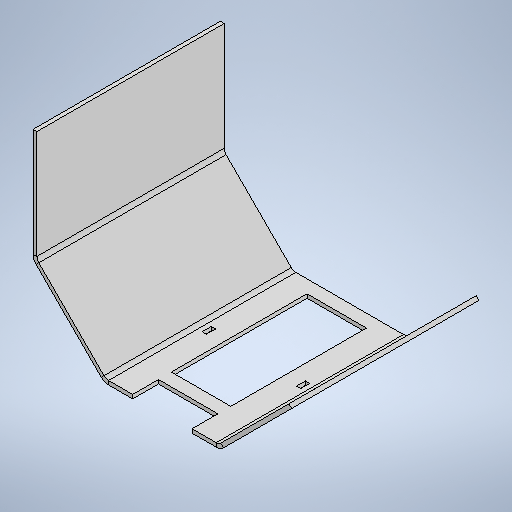
# Autodesk Inventor part: DSB-101 Axis
Saved by Autodesk Inventor 2025.1 (Build 291241020, 241B)
## iProperties
Created: 2025-01-13
Part Number: DSB-101 Axis
Material: Stainless Steel
Document SubType Name: Sheet Metal
Designer: Dobrov
Mass: 256.049 g
Surface Area: 335.823 cm^2
Volume: 32.0061 cm^3
Density: 8 g/cm^3
Sheet Metal Rule: AISI304 3mm Die 32
Sheet Metal Width: 145.000 mm
Sheet Metal Length: 328.009 mm
Sheet Metal Area: 47561.290 mm^2
Appearance: Default
Flat Pattern Width: 14.5 cm
Flat Pattern Length: 32.8009 cm
Flat Pattern Area: 475.613 cm^2
Author: user
Autodesk Inventor part; units mm, degrees
ref_plane "YZ Plane" through (0, 0, 0) normal (1, 0, 0) x (0, 1, 0)
ref_plane "XZ Plane" through (0, 0, 0) normal (0, 1, 0) x (-1, 0, 0)
ref_plane "XY Plane" through (0, 0, 0) normal (0, 0, 1) x (1, 0, 0)
sketch "Sketch1" plane through (0, 0, 0) normal (0, 0, 1) x (1, 0, 0)
  line L0 (-45, -72.5) -> (45, -72.5)
  line L1 (45, -72.5) -> (45, 72.5)
  line L2 (45, 72.5) -> (-45, 72.5)
  line L3 (-45, 72.5) -> (-45, -72.5)
  line L4 (-45, -72.5) -> (45, 72.5) construction
  line L5 (45, -72.5) -> (-45, 72.5) construction
  point P0 (0, 0)
  dimension "d154" = 90
  dimension "d155" = 145
  measures "d154" distance of L1.end L2.end
  measures "d155" distance of L0.end L1.end
extrude "Plate3" add sketch "Sketch1" along normal blind 3
sketch "Sketch7" plane through (42.8787, 72.5, 2.1213) normal (0.7071068, 0, -0.7071068) x (0, 1, 0)
  line L0 (-145, 0) -> (0, 0)
  line L1 (0, 0) -> (0, 78)
  line L2 (0, 78) -> (-145, 78)
  line L3 (-145, 78) -> (-145, 0)
  constraints: 6 end point, 1 horizontal, 1 perpendicular, 1 vertical
edge flange "Flange3" height 78 angle 45 thickness 3 bend radius 5 thickness toward (0.7071068, 0, -0.7071068) relief round relief width 3 relief depth 1.5 corner gap 5 corner form 0 edges at (45, 0, 3) (-45, 0, 3) wall of the first edge with corners at (42.8787, -72.5, 2.1213) (42.8787, 72.5, 2.1213) (98.033, 72.5, 57.2756) (98.033, -72.5, 57.2756)
bend "Bend3"
corner "Corner3"
sketch "Sketch8" plane through (0, 0, 3) normal (0, 0, 1) x (1, 0, 0)
  line L0 (23, 62.5) -> (-23, 62.5)
  line L1 (-23, 62.5) -> (-23, -42.5)
  line L2 (-23, -42.5) -> (23, -42.5)
  line L3 (23, -42.5) -> (23, 62.5)
  line L4 (23, 62.5) -> (-23, -42.5) construction
  line L5 (-23, 62.5) -> (23, -42.5) construction
  line L6 (-45, 72.5) -> (41.6863, 72.5) projected
  line L7 (-41.6863, -72.5) -> (41.6863, -72.5) projected
  line L8 (23, -72.5) -> (-23, -72.5)
  line L9 (-23, -72.5) -> (-23, -52.5)
  line L10 (-23, -52.5) -> (23, -52.5)
  line L11 (23, -52.5) -> (23, -72.5)
  point P0 (0, 0)
  point P1 (0, 10)
  point P2 (-23, -72.5)
  point P3 (33.1873, -84)
  dimension "d166" = 46
  dimension "d168" = 10
  dimension "d182" = 10
  dimension "d183" = 20
  constraints: 20 end point, 4 parallel, 2 collinear, 2 horizontal, 2 midpoint, 2 perpendicular, 1 point on line, 1 vertical alignment
  measures "d166" distance of L2.end L1.end
  measures "d168" distance between parallel lines of L0 L6
  measures "d182" distance between parallel lines of L10 L2
  measures "d183" distance of L8.end L9.end
extrude "Cut1" cut sketch "Sketch8" against normal blind 3
sketch "Sketch9" plane through (-97.1543, -72.5, 55.1543) normal (-1, 0, 0) x (0, -1, 0)
  line L0 (-145, 0) -> (0, 0)
  line L1 (0, 0) -> (0, 87)
  line L2 (0, 87) -> (-145, 87)
  line L3 (-145, 87) -> (-145, 0)
  constraints: 6 end point, 1 horizontal, 1 perpendicular, 1 vertical
edge flange "Flange4" height 87 angle 45 thickness 3 bend radius 5 thickness toward (-1, 0, 0) relief round relief width 3 relief depth 1.5 edges at (-98.033, 0, 57.2756) wall of the first edge with corners at (-97.1543, 72.5, 55.1543) (-97.1543, -72.5, 55.1543) (-97.1543, -72.5, 142.1543) (-97.1543, 72.5, 142.1543)
bend "Bend4"
corner "Corner4"
sketch "Sketch10" plane through (0, 0, 3) normal (0, 0, 1) x (1, 0, 0)
  line L0 (-38.15, 3.5) -> (-34.85, 3.5)
  line L1 (-34.85, 3.5) -> (-34.85, -3.5)
  line L2 (-34.85, -3.5) -> (-38.15, -3.5)
  line L3 (-38.15, -3.5) -> (-38.15, 3.5)
  line L4 (-38.15, 3.5) -> (-34.85, -3.5) construction
  line L5 (-34.85, 3.5) -> (-38.15, -3.5) construction
  line L6 (34.85, 3.5) -> (38.15, 3.5)
  line L7 (38.15, 3.5) -> (38.15, -3.5)
  line L8 (38.15, -3.5) -> (34.85, -3.5)
  line L9 (34.85, -3.5) -> (34.85, 3.5)
  line L10 (34.85, 3.5) -> (38.15, -3.5) construction
  line L11 (38.15, 3.5) -> (34.85, -3.5) construction
  line L12 (0, 0) -> (0, 29.0693)
  line L13 (41.6863, -72.5) -> (23, -72.5) projected
  point P0 (-36.5, 0)
  point P1 (36.5, 0)
  point P2 (-36.5, 3.5)
  point P3 (36.5, 3.5)
  dimension "d184" = 7
  dimension "d185" = 3.3
  dimension "d186" = 69
  dimension "d187" = 73
  constraints: 26 end point, 6 midpoint, 4 parallel, 2 equal length, 2 horizontal, 2 perpendicular, 1 horizontal alignment, 1 vertical, 1 other
  measures "d184" distance of L8.end L6.start
  measures "d185" distance of L6.start L6.end
  measures "d186" distance between parallel lines of L8 L13
  measures "d187" distance of point (36.5, 0) point (-36.5, 0)
extrude "Cut2" cut sketch "Sketch10" against normal blind 3
body "Solid2"
